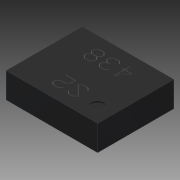
# Autodesk Inventor part: LSM6DS3 Accelerometer
Saved by Autodesk Inventor 2016 (Build 200138000, 138)
## iProperties
Created: 2019-08-17
Part Number: LSM6DS3 Accelerometer
Material: Silicon Nitride
Document SubType Name: Modeling
Designer: Orest
Mass: 0.0199407 g
Surface Area: 0.248311 cm^2
Volume: 0.00627067 cm^3
Density: 3.18 g/cm^3
Appearance: Smooth - Black (BGA)
Catalog Web Link: https://www.st.com/content/ccc/resource/technical/document/datasheet/a3/f5/4f/ae/8e/44/41/d7/DM00133076.pdf/files/DM00133076.pdf/jcr:content/translations/en.DM00133076.pdf
Author: Orest
Autodesk Inventor part; units mm, degrees
ref_plane "YZ Plane" through (0, 0, 0) normal (1, 0, 0) x (0, 1, 0)
ref_plane "XZ Plane" through (0, 0, 0) normal (0, 1, 0) x (-1, 0, 0)
ref_plane "XY Plane" through (0, 0, 0) normal (0, 0, 1) x (1, 0, 0)
sketch "Sketch10" plane through (0, 0, 0) normal (0, 1, 0) x (-1, 0, 0)
  line L0 (1.25, 1.5) -> (-1.25, 1.5)
  line L1 (-1.25, 1.5) -> (-1.25, -1.5)
  line L2 (-1.25, -1.5) -> (1.25, -1.5)
  line L3 (1.25, -1.5) -> (1.25, 1.5)
  point P0 (0, 0)
  point P1 (1.25, 0)
  point P2 (0, 1.5)
  dimension "d7" = 2.5
  dimension "d8" = 3
  constraints: 8 end point, 2 midpoint, 2 parallel, 1 horizontal, 1 horizontal alignment, 1 perpendicular, 1 vertical alignment
  measures "d7" distance of L2.end L1.end
  measures "d8" distance of L1.end L0.end
extrude "Extrusion4" add sketch "Sketch10" along normal blind 0.83
sketch "Sketch11" plane through (0, 0.83, 0) normal (0, 1, 0) x (1, 0, 0)
  line L0 (0.875, -0.5) -> (0.875, 0.5) construction
  line L1 (0.875, 0.5) -> (-0.875, 0.5) construction
  line L2 (-0.875, 0.5) -> (-0.875, -0.5) construction
  line L3 (-0.875, -0.5) -> (0.875, -0.5) construction
  line L4 (-1.25, -1.5) -> (1.25, -1.5) projected
  line L5 (1.25, -1.5) -> (1.25, 1.5) projected
  line L6 (1.25, 1.5) -> (-1.25, 1.5) projected
  line L7 (-1.25, 1.5) -> (-1.25, -1.5) projected
  circle A0 centre (-0.75, -1) radius 0.2
  line L8 (-0.4729, -0.0698) -> (-0.3802, -0.1604)
  line L9 (-0.3802, -0.1604) -> (-0.3802, -0.3325)
  line L10 (-0.3802, -0.3325) -> (-0.4691, -0.4194)
  line L11 (-0.4691, -0.4194) -> (-0.4838, -0.4048)
  line L12 (-0.4838, -0.4048) -> (-0.404, -0.3229)
  line L13 (-0.404, -0.3229) -> (-0.404, -0.1704)
  line L14 (-0.404, -0.1704) -> (-0.4729, -0.0986)
  line L15 (-0.4729, -0.0986) -> (-0.7971, -0.4227)
  line L16 (-0.7971, -0.4227) -> (-0.8902, -0.3325)
  line L17 (-0.8902, -0.3325) -> (-0.8902, -0.1604)
  line L18 (-0.8902, -0.1604) -> (-0.8012, -0.0735)
  line L19 (-0.8012, -0.0735) -> (-0.7866, -0.0886)
  line L20 (-0.7866, -0.0886) -> (-0.8664, -0.1708)
  line L21 (-0.8664, -0.1708) -> (-0.8664, -0.3225)
  line L22 (-0.8664, -0.3225) -> (-0.7971, -0.3943)
  line L23 (-0.7971, -0.3943) -> (-0.4729, -0.0698)
  line L24 (-0.7114, 0.4248) -> (-0.6229, 0.3363)
  line L25 (-0.6229, 0.3363) -> (-0.6229, 0.1742)
  line L26 (-0.6229, 0.1742) -> (-0.5493, 0.1007)
  line L27 (-0.5493, 0.1007) -> (-0.404, 0.1007)
  line L28 (-0.404, 0.1007) -> (-0.404, 0.419)
  line L29 (-0.404, 0.419) -> (-0.3802, 0.419)
  line L30 (-0.3802, 0.419) -> (-0.3802, 0.076)
  line L31 (-0.3802, 0.076) -> (-0.559, 0.076)
  line L32 (-0.559, 0.076) -> (-0.6471, 0.1642)
  line L33 (-0.6471, 0.1642) -> (-0.6471, 0.3262)
  line L34 (-0.6471, 0.3262) -> (-0.721, 0.4002)
  line L35 (-0.721, 0.4002) -> (-0.792, 0.4002)
  line L36 (-0.792, 0.4002) -> (-0.8664, 0.3258)
  line L37 (-0.8664, 0.3258) -> (-0.8664, 0.1742)
  line L38 (-0.8664, 0.1742) -> (-0.7866, 0.0919)
  line L39 (-0.7866, 0.0919) -> (-0.8012, 0.0773)
  line L40 (-0.8012, 0.0773) -> (-0.8902, 0.1642)
  line L41 (-0.8902, 0.1642) -> (-0.8902, 0.3363)
  line L42 (-0.8902, 0.3363) -> (-0.8016, 0.4248)
  line L43 (-0.8016, 0.4248) -> (-0.7114, 0.4248)
  line L44 (0.7281, -0.326) -> (0.7281, -0.4012)
  line L45 (0.7281, -0.4012) -> (0.8852, -0.4012)
  line L46 (0.8852, -0.4012) -> (0.8852, -0.4259)
  line L47 (0.8852, -0.4259) -> (0.7281, -0.4259)
  line L48 (0.7281, -0.4259) -> (0.7281, -0.6748)
  line L49 (0.7281, -0.6748) -> (0.3693, -0.4012)
  line L50 (0.3693, -0.4012) -> (0.7043, -0.4012)
  line L51 (0.7043, -0.4012) -> (0.7043, -0.326)
  line L52 (0.7043, -0.326) -> (0.7281, -0.326)
  line L53 (0.7043, -0.4259) -> (0.4148, -0.4259)
  line L54 (0.4148, -0.4259) -> (0.7043, -0.6393)
  line L55 (0.7043, -0.6393) -> (0.7043, -0.4259)
  line L56 (0.8021, 0.1765) -> (0.8902, 0.0879)
  line L57 (0.8902, 0.0879) -> (0.8902, -0.0842)
  line L58 (0.8902, -0.0842) -> (0.8012, -0.1711)
  line L59 (0.8012, -0.1711) -> (0.7866, -0.1564)
  line L60 (0.7866, -0.1564) -> (0.8664, -0.0746)
  line L61 (0.8664, -0.0746) -> (0.8664, 0.0779)
  line L62 (0.8664, 0.0779) -> (0.7925, 0.1518)
  line L63 (0.7925, 0.1518) -> (0.721, 0.1518)
  line L64 (0.721, 0.1518) -> (0.6475, 0.0775)
  line L65 (0.6475, 0.0775) -> (0.6475, -0.0048)
  line L66 (0.6475, -0.0048) -> (0.6233, -0.0048)
  line L67 (0.6233, -0.0048) -> (0.6233, 0.0779)
  line L68 (0.6233, 0.0779) -> (0.5493, 0.1518)
  line L69 (0.5493, 0.1518) -> (0.4783, 0.1518)
  line L70 (0.4783, 0.1518) -> (0.404, 0.0775)
  line L71 (0.404, 0.0775) -> (0.404, -0.0741)
  line L72 (0.404, -0.0741) -> (0.4838, -0.1564)
  line L73 (0.4838, -0.1564) -> (0.4691, -0.1711)
  line L74 (0.4691, -0.1711) -> (0.3802, -0.0842)
  line L75 (0.3802, -0.0842) -> (0.3802, 0.0879)
  line L76 (0.3802, 0.0879) -> (0.4687, 0.1765)
  line L77 (0.4687, 0.1765) -> (0.559, 0.1765)
  line L78 (0.559, 0.1765) -> (0.6354, 0.0971)
  line L79 (0.6354, 0.0971) -> (0.7118, 0.1765)
  line L80 (0.7118, 0.1765) -> (0.8021, 0.1765)
  line L81 (0.8021, 0.6731) -> (0.8902, 0.5846)
  line L82 (0.8902, 0.5846) -> (0.8902, 0.4125)
  line L83 (0.8902, 0.4125) -> (0.8025, 0.3244)
  line L84 (0.8025, 0.3244) -> (0.7114, 0.3244)
  line L85 (0.7114, 0.3244) -> (0.6354, 0.4029)
  line L86 (0.6354, 0.4029) -> (0.5594, 0.3244)
  line L87 (0.5594, 0.3244) -> (0.4683, 0.3244)
  line L88 (0.4683, 0.3244) -> (0.3802, 0.4125)
  line L89 (0.3802, 0.4125) -> (0.3802, 0.5846)
  line L90 (0.3802, 0.5846) -> (0.4687, 0.6731)
  line L91 (0.4687, 0.6731) -> (0.559, 0.6731)
  line L92 (0.559, 0.6731) -> (0.6354, 0.5938)
  line L93 (0.6354, 0.5938) -> (0.7118, 0.6731)
  line L94 (0.7118, 0.6731) -> (0.8021, 0.6731)
  line L95 (0.5493, 0.6485) -> (0.4779, 0.6485)
  line L96 (0.4779, 0.6485) -> (0.404, 0.5741)
  line L97 (0.404, 0.5741) -> (0.404, 0.4225)
  line L98 (0.404, 0.4225) -> (0.4779, 0.349)
  line L99 (0.4779, 0.349) -> (0.5493, 0.349)
  line L100 (0.5493, 0.349) -> (0.6233, 0.4221)
  line L101 (0.6233, 0.4221) -> (0.6233, 0.5746)
  line L102 (0.6233, 0.5746) -> (0.5493, 0.6485)
  line L103 (0.7925, 0.6485) -> (0.721, 0.6485)
  line L104 (0.721, 0.6485) -> (0.6475, 0.5741)
  line L105 (0.6475, 0.5741) -> (0.6475, 0.4225)
  line L106 (0.6475, 0.4225) -> (0.721, 0.349)
  line L107 (0.721, 0.349) -> (0.7929, 0.349)
  line L108 (0.7929, 0.349) -> (0.8664, 0.4221)
  line L109 (0.8664, 0.4221) -> (0.8664, 0.5746)
  line L110 (0.8664, 0.5746) -> (0.7925, 0.6485)
  point P0 (0, 0)
  point P1 (-0.875, 0)
  point P2 (-1.25, 0)
  point P3 (0, -0.5)
  point P4 (0, -1.5)
  dimension "d11" = 1.75
  dimension "d12" = 1
  dimension "d13" = 0.4
  dimension "d14" = 0.5
  dimension "d15" = 0.5
  constraints: 4 midpoint, 1 centre point, 1 horizontal alignment, 1 vertical, 1 vertical alignment, 2 other
  measures "d11" distance between parallel lines of L0 L2
  measures "d12" distance between parallel lines of L1 L3
  measures "d13" diameter of A0
  measures "d14" distance from line of L4 A0.centre
  measures "d15" distance from line of L7 A0.centre
extrude "Extrusion5" cut sketch "Sketch11" against normal blind 0.01 contours L8 L9 L10 L11 L12 L13 L14 L15 L16 L17 L18 L19 L20 L21 L22 L23 | L24 L25 L26 L27 L28 L29 L30 L31 L32 L33 L34 L35 L36 L37 L38 L39 L40 L41 L42 L43 | L44 L45 L46 L47 L48 L49 L50 L51 L52 | L56 L57 L58 L59 L60 L61 L62 L63 L64 L65 L66 L67 L68 L69 L70 L71 L72 L73 L74 L75 L76 L77 L78 L79 L80 | L81 L82 L83 L84 L85 L86 L87 L88 L89 L90 L91 L92 L93 L94
extrude "Extrusion6" cut sketch "Sketch11" against normal blind 0.05 contours A0
sketch "Sketch12" plane through (0, 0, 0) normal (0, -1, 0) x (1, 0, 0)
  line L0 (-1.15, -0.675) -> (-0.6, -0.675)
  line L1 (-0.6, -0.675) -> (-0.6, -0.325)
  line L2 (-0.6, -0.325) -> (-1.15, -0.325)
  line L3 (-1.15, -0.325) -> (-1.15, -0.675)
  line L4 (-1.25, 1.5) -> (1.25, 1.5) construction
  line L5 (-1.25, -1.5) -> (-1.25, 1.5) construction
  line L6 (1.25, -1.5) -> (-1.25, -1.5) construction
  line L7 (1.25, 1.5) -> (1.25, -1.5) construction
  line L8 (-1.15, -0.175) -> (-0.6, -0.175)
  line L9 (-0.6, -0.175) -> (-0.6, 0.175)
  line L10 (-0.6, 0.175) -> (-1.15, 0.175)
  line L11 (-1.15, 0.175) -> (-1.15, -0.175)
  line L12 (-1.15, 0.325) -> (-0.6, 0.325)
  line L13 (-0.6, 0.325) -> (-0.6, 0.675)
  line L14 (-0.6, 0.675) -> (-1.15, 0.675)
  line L15 (-1.15, 0.675) -> (-1.15, 0.325)
  line L16 (-0.575, -1.4) -> (-0.925, -1.4)
  line L17 (-0.925, -1.4) -> (-0.925, -0.85)
  line L18 (-0.925, -0.85) -> (-0.575, -0.85)
  line L19 (-0.575, -0.85) -> (-0.575, -1.4)
  line L20 (-0.425, -1.4) -> (-0.425, -0.85)
  line L21 (-0.075, -1.4) -> (-0.425, -1.4)
  line L22 (-0.075, -0.85) -> (-0.075, -1.4)
  line L23 (-0.425, -0.85) -> (-0.075, -0.85)
  line L24 (0.075, -1.4) -> (0.075, -0.85)
  line L25 (0.425, -1.4) -> (0.075, -1.4)
  line L26 (0.425, -0.85) -> (0.425, -1.4)
  line L27 (0.075, -0.85) -> (0.425, -0.85)
  line L28 (0.575, -1.4) -> (0.575, -0.85)
  line L29 (0.925, -1.4) -> (0.575, -1.4)
  line L30 (0.925, -0.85) -> (0.925, -1.4)
  line L31 (0.575, -0.85) -> (0.925, -0.85)
  line L32 (-1.25, 0) -> (1.25, 0) construction
  line L33 (0, 1.5) -> (0, -1.5) construction
  line L34 (1.15, -0.675) -> (0.6, -0.675)
  line L35 (0.6, -0.675) -> (0.6, -0.325)
  line L36 (0.6, -0.325) -> (1.15, -0.325)
  line L37 (1.15, -0.325) -> (1.15, -0.675)
  line L38 (1.15, -0.175) -> (0.6, -0.175)
  line L39 (0.6, -0.175) -> (0.6, 0.175)
  line L40 (0.6, 0.175) -> (1.15, 0.175)
  line L41 (1.15, 0.175) -> (1.15, -0.175)
  line L42 (1.15, 0.325) -> (0.6, 0.325)
  line L43 (0.6, 0.325) -> (0.6, 0.675)
  line L44 (0.6, 0.675) -> (1.15, 0.675)
  line L45 (1.15, 0.675) -> (1.15, 0.325)
  line L46 (-0.575, 1.4) -> (-0.925, 1.4)
  line L47 (-0.925, 1.4) -> (-0.925, 0.85)
  line L48 (-0.925, 0.85) -> (-0.575, 0.85)
  line L49 (-0.575, 0.85) -> (-0.575, 1.4)
  line L50 (-0.425, 1.4) -> (-0.425, 0.85)
  line L51 (-0.075, 1.4) -> (-0.425, 1.4)
  line L52 (-0.075, 0.85) -> (-0.075, 1.4)
  line L53 (-0.425, 0.85) -> (-0.075, 0.85)
  line L54 (0.075, 1.4) -> (0.075, 0.85)
  line L55 (0.425, 1.4) -> (0.075, 1.4)
  line L56 (0.425, 0.85) -> (0.425, 1.4)
  line L57 (0.075, 0.85) -> (0.425, 0.85)
  line L58 (0.575, 1.4) -> (0.575, 0.85)
  line L59 (0.925, 1.4) -> (0.575, 1.4)
  line L60 (0.925, 0.85) -> (0.925, 1.4)
  line L61 (0.575, 0.85) -> (0.925, 0.85)
  line L62 (0.075, -0.85) -> (-0.075, -0.85) construction
  line L63 (-1.25, -1.5) -> (-1.25, 1.5) construction
  point P0 (0, 0)
  point P1 (-0.6, 0)
  point P2 (0, -0.85)
  dimension "d22" = 0.5
  dimension "d29" = 0.5
  dimension "d36" = 0.1
  dimension "d37" = 0.1
  dimension "d38" = 0.55
  dimension "d39" = 0.35
  constraints: 118 end point, 28 symmetric about line, 6 midpoint, 4 horizontal, 4 parallel, 4 perpendicular, 2 point on line, 1 vertical, 40 other
  measures "d22" distance of L0.start L8.start
  measures "d29" distance of L17.end L20.end
  measures "d36" distance between parallel lines of L6 L16
  measures "d37" distance between parallel lines of L5 L15
  measures "d38" distance of L30.start L29.start
  measures "d39" distance between parallel lines of L36 L34
extrude "Extrusion7" add sketch "Sketch12" along normal blind 0.02
chamfer "Chamfer1" distance 0.2 angle 45 1 edges at (-0.925, -0.01, 0.85)
equation "\"d29\" = d22"
equation "\"d37\" = d36"
body "Solid4"
